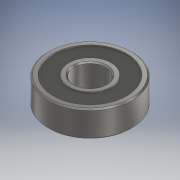
# Autodesk Inventor part: 6201-2RS
Saved by Autodesk Inventor 2017 (Build 210142000, 142)
## iProperties
Created: 2019-10-31
Part Number: 6201-2RS
Material: Stainless Steel
Document SubType Name: Modeling
Designer: Dell
Density: 8 g/cm^3
Appearance: Semi-Polished
Author: Dell
Autodesk Inventor part; units mm, degrees
ref_plane "YZ Plane" through (0, 0, 0) normal (1, 0, 0) x (0, 1, 0)
ref_plane "XZ Plane" through (0, 0, 0) normal (0, 1, 0) x (-1, 0, 0)
ref_plane "XY Plane" through (0, 0, 0) normal (0, 0, 1) x (1, 0, 0)
sketch "Sketch1" plane through (0, 0, 0) normal (0, 0, 1) x (1, 0, 0)
  circle A0 centre (0, 0) radius 6
  circle A1 centre (0, 0) radius 16
  dimension "d0" = 12
  dimension "d1" = 32
  constraints: 2 centre point, 2 coincident
  measures "d0" diameter of A0
  measures "d1" diameter of A1
extrude "Extrusion1" add sketch "Sketch1" along normal blind 10
sketch "Sketch2" plane through (0, 0, 10) normal (0, 0, 1) x (1, 0, 0)
  circle A0 centre (0, 0) radius 6 projected
  circle A1 centre (0, 0) radius 6 projected
  circle A2 centre (0, 0) radius 16 projected
  circle A3 centre (0, 0) radius 8
  circle A4 centre (0, 0) radius 14
  dimension "d4" = 2
  dimension "d5" = 2
  constraints: 2 centre point
  measures "d4" radial gap between concentric circles of A0 A3
  measures "d5" radial gap between concentric circles of A2 A4
extrude "Extrusion2" cut sketch "Sketch2" against normal blind 0.5 contours A4
sketch "Sketch3" plane through (0, 0, 0) normal (0, 0, -1) x (-1, 0, 0)
  circle A0 centre (0, 0) radius 8 projected
  circle A1 centre (0, 0) radius 14 projected
extrude "Extrusion3" cut sketch "Sketch3" against normal blind 0.5
chamfer "Chamfer1" distance 0.5 angle 45 4 edges at (-16, 0, 10) (-16, 0, 0) (-6, 0, 10) (-6, 0, 0)
body "Solid1"
